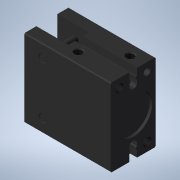
# Autodesk Inventor part: MCHA-20_(b)
Saved by Autodesk Inventor 2021 (Build 250183000, 183)
## iProperties
Created: 2025-07-26
Part Number: MCHA-20_(b)
Material: Generic
Catalog Web Link: www.cadenas.de
Description: MCHA-body-Grippers
Vendor: MINDMAN
Document SubType Name: Modeling
Designer: psAdmin
Manufacturer: MINDMAN
Mass: 44.4877 g
Surface Area: 130.835 cm^2
Volume: 44.4877 cm^3
Density: 1 g/cm^3
Appearance: PSOLRGB-175-175-175
Category: PARTsolutions
Company: MINDMAN
Title: MCHA-20_(b)
Author: Cadenas PARTsolutions
Comments: Grippers
PSOL_IDENT_0: {$CADENAS_DATA/23d-libs/mindman/end_of_arm_tooling/grippers/angular_gripper/mcha/mcha_body.prj},177
PSOL_IDENT_1: {VTYP=3D},{NB=MCHA-20_(b)},{LINA=MCHA-20_(b)},{NN=MCHA-body},{DATE=13.05.2025 08:42:05},{GEOMDATE=13
PSOL_IDENT_2: .05.2025 08:42:00},{VERSION=},{LINEID=30},{WBVAR=MODEL,SWITCH},{WBNUMERIC=}  {NB=MCHA-20_(b)},{LINA=
PSOL_IDENT_3: MCHA-20_(b)},{KT=DUMMY},{IDNR=MIN},{CODE=MCHA-20},{MODEL=MCHA},{TUBE=20},{A=22.0},{B=4},{C=10},{D=12
PSOL_IDENT_4: },{E=40.1},{F=18},{G=30},{H=8.0},{I=13.0},{J=25.0},{K=45},{L=25.0},{M=39.5},{N=32.5},{O=16.0},{P=19.
PSOL_IDENT_5: 0},{Q=50.0},{R=16},{S=26},{T=35},{UU=M5 x 8depth},{VV=M5 x 8depth},{WW=M5 x 12depth},{XX=M5 x 5depth
PSOL_IDENT_6: },{YY=M4},{Z=7},{ZZ=3.5},{A1=29.2},{B1=0.0},{C1=0.1},{A2=29.2},{B2=1.9},{C2=0.0},{SWITCH=},{XSWITCH=''
PSOL_IDENT_7: ,'Blank: without switch','+RCE','RCE : 2 wire (Reed switch)','+RDE','RDE : 2 wire (Non+contact)','+R
PSOL_IDENT_8: DE-D','RDE-D : 2 wire (Non+contact)','+RNE','RNE : 3 wire(NPN current sinking)','+RNEE','RNEE : 3 wi
PSOL_IDENT_9: re(NPN current sinking)','+RPE','RPE : 3 wire(PNP current sourcing)','+RPEE','RPEE : 3 wire(PNP curr
PSOL_IDENT_10: ent sourcing)'}
NB: MCHA-20_(b)
NN: MCHA-body
NT: Grippers
NBSYN: $CODE._(b)
LINA: MCHA-20_(b)
CATALOG: MINDMAN
MODEL: MCHA
TUBE: 20
A: 22
B: 4
C: 10
D: 12
E: 40.1
F: 18
G: 30
H: 8
I: 13
J: 25
K: 45
L: 25
M: 39.5
N: 32.5
O: 16
P: 19
Q: 50
R: 16
S: 26
T: 35
UU: M5 x 8depth
VV: M5 x 8depth
WW: M5 x 12depth
XX: M5 x 5depth
YY: M4
Z: 7
ZZ: 3.5
A1: 29.2
B1: 0
C1: 0.1
A2: 29.2
B2: 1.9
C2: 0
SWITCH: Blank: without switch
SUPPLIER: MINDMAN
ARTICLENO: MCHA-20_(b)
BOMINFO: MCHA-20_(b)
CREATOR: CADENAS GmbH
Autodesk Inventor part; units mm, degrees
sketch "Sketch_1" plane through (0, 0, 0) normal (1, 0, 0) x (0, 1, 0)
  line L0 (-22, 13) -> (-22.5, 12.5)
  line L1 (-22.5, 12.5) -> (-22.5, 2.25)
  line L2 (-22.5, 2.25) -> (-18.5, 2.25)
  line L3 (-18.5, 2.25) -> (-18.5, 1.9)
  arc A0 (-18.5, 1.9) -> (-18.3, 1.7) centre (-18.3, 1.9) ccw
  line L4 (-18.3, 1.7) -> (-17, 1.7)
  line L5 (-17, 1.7) -> (-16.5, 2.15)
  line L6 (-16.5, 2.15) -> (-14.7, 2.15)
  arc A1 (-13, 0.45) -> (-14.7, 2.15) centre (-14.7, 0.45) ccw
  line L7 (-13, 0.45) -> (-13, -0.45)
  arc A2 (-14.7, -2.15) -> (-13, -0.45) centre (-14.7, -0.45) ccw
  line L8 (-14.7, -2.15) -> (-16.5, -2.15)
  line L9 (-16.5, -2.15) -> (-17, -1.7)
  line L10 (-17, -1.7) -> (-18.3, -1.7)
  arc A3 (-18.3, -1.7) -> (-18.5, -1.9) centre (-18.3, -1.9) ccw
  line L11 (-18.5, -1.9) -> (-18.5, -2.25)
  line L12 (-18.5, -2.25) -> (-22.5, -2.25)
  line L13 (-22.5, -2.25) -> (-22.5, -12.5)
  line L14 (-22.5, -12.5) -> (-22, -13)
  line L15 (-22, -13) -> (22, -13)
  line L16 (22, -13) -> (22.5, -12.5)
  line L17 (22.5, -12.5) -> (22.5, -2.25)
  line L18 (22.5, -2.25) -> (18.5, -2.25)
  line L19 (18.5, -2.25) -> (18.5, -1.9)
  arc A4 (18.5, -1.9) -> (18.3, -1.7) centre (18.3, -1.9) ccw
  line L20 (18.3, -1.7) -> (17, -1.7)
  line L21 (17, -1.7) -> (16.5, -2.15)
  line L22 (16.5, -2.15) -> (14.7, -2.15)
  arc A5 (13, -0.45) -> (14.7, -2.15) centre (14.7, -0.45) ccw
  line L23 (13, -0.45) -> (13, 0.45)
  arc A6 (14.7, 2.15) -> (13, 0.45) centre (14.7, 0.45) ccw
  line L24 (14.7, 2.15) -> (16.5, 2.15)
  line L25 (16.5, 2.15) -> (17, 1.7)
  line L26 (17, 1.7) -> (18.3, 1.7)
  arc A7 (18.3, 1.7) -> (18.5, 1.9) centre (18.3, 1.9) ccw
  line L27 (18.5, 1.9) -> (18.5, 2.25)
  line L28 (18.5, 2.25) -> (22.5, 2.25)
  line L29 (22.5, 2.25) -> (22.5, 12.5)
  line L30 (22.5, 12.5) -> (22, 13)
  line L31 (22, 13) -> (-22, 13)
  constraints: 64 end point, 16 point on circle, 8 centre point
extrude "Extrusion1" add sketch "Sketch_1" along normal blind 50
sketch "Sketch2" plane through (50, 0, 0) normal (1, 0, 0) x (0, 0, -1)
  point P0 (0, 0)
hole "Hole1" at (50, 0, 0) direction (-1, 0, 0) diameter 22 depth 1.5
sketch "Sketch3" plane through (50, 0, 0) normal (1, 0, 0) x (0, 0, -1)
  point P0 (8, 17.5)
hole "Hole2" at (50, 17.5, -8) direction (-1, 0, 0) diameter 4 depth 4
sketch "Sketch_3" plane through (0, 0, 0) normal (0, 1, 0) x (-1, 0, 0)
  line L0 (0, 6.05) -> (-18.5, 6.05)
  line L1 (-18.5, 6.05) -> (-18.5, -6.05)
  line L2 (-18.5, -6.05) -> (0, -6.05)
  line L3 (0, -6.05) -> (0, 6.05)
  constraints: 8 end point
extrude "Extrusion2" cut sketch "Sketch_3" along normal mid plane 60
sketch "Sketch5" plane through (50, 0, 0) normal (1, 0, 0) x (0, 0, -1)
  point P0 (8, -17.5)
hole "Hole3" at (50, -17.5, -8) direction (-1, 0, 0) diameter 4.134 depth 11 tip angle 120 countersink diameter 5 countersink angle 90 thread size "M5x0.8" class "6H" standard "ISO Metric profile"
sketch "Sketch6" plane through (50, 0, 0) normal (1, 0, 0) x (0, 0, -1)
  point P0 (-8, 17.5)
hole "Hole4" at (50, 17.5, 8) direction (-1, 0, 0) diameter 4.134 depth 11 tip angle 120 countersink diameter 5 countersink angle 90 thread size "M5x0.8" class "6H" standard "ISO Metric profile"
sketch "Sketch_6" plane through (0, 0, 6.5) normal (0, 0, 1) x (1, 0, 0)
  line L0 (25, 6.3066) -> (25, 22.5)
  line L1 (25, 22.5) -> (27.5, 22.5)
  line L2 (27.5, 22.5) -> (27.067, 22.067)
  line L3 (27.067, 22.067) -> (27.067, 15.5)
  line L4 (27.067, 15.5) -> (25.75, 14.7396)
  line L5 (25.75, 14.7396) -> (25.75, 6.7396)
  line L6 (25.75, 6.7396) -> (25, 6.3066)
  line L7 (25, 6.3066) -> (25, 22.5)
  constraints: 16 end point
revolve "Revolution1" cut sketch "Sketch_6" angle 360 about axis through (25, 6.3066, 6.5) along (0, -1, 0)
thread "Thread1" size "M5x0.8" class "6H" standard "ISO Metric profile" length 4.567
sketch "Sketch_7" plane through (0, 0, -6.5) normal (0, 0, 1) x (1, 0, 0)
  line L0 (42, 6.3066) -> (42, 22.5)
  line L1 (42, 22.5) -> (44.5, 22.5)
  line L2 (44.5, 22.5) -> (44.067, 22.067)
  line L3 (44.067, 22.067) -> (44.067, 15.5)
  line L4 (44.067, 15.5) -> (42.75, 14.7396)
  line L5 (42.75, 14.7396) -> (42.75, 6.7396)
  line L6 (42.75, 6.7396) -> (42, 6.3066)
  line L7 (42, 6.3066) -> (42, 22.5)
  constraints: 16 end point
revolve "Revolution2" cut sketch "Sketch_7" angle 360 about axis through (42, 6.3066, -6.5) along (0, -1, 0)
thread "Thread2" size "M5x0.8" class "6H" standard "ISO Metric profile" length 4.567
sketch "Sketch9" plane through (0, -22.5, 12.5) normal (0, -1, 0) x (1, 0, 0)
  point P0 (31, -4.5)
hole "Hole5" at (31, -22.5, 8) direction (0, 1, 0) diameter 4.134 depth 11 tip angle 120 countersink diameter 5 countersink angle 90 thread size "M5x0.8" class "6H" standard "ISO Metric profile"
sketch "Sketch10" plane through (0, -22.5, -12.5) normal (0, -1, 0) x (1, 0, 0)
  point P0 (31, 4.5)
hole "Hole6" at (31, -22.5, -8) direction (0, 1, 0) diameter 4.134 depth 11 tip angle 120 countersink diameter 5 countersink angle 90 thread size "M5x0.8" class "6H" standard "ISO Metric profile"
sketch "Sketch11" plane through (0, -22, -13) normal (0, 0, -1) x (-1, 0, 0)
  point P0 (-25, 7)
hole "Hole7" at (25, -15, -13) direction (0, 0, 1) diameter 4.134 depth 12 tip angle 120 countersink diameter 5 countersink angle 90 thread size "M5x0.8" class "6H" standard "ISO Metric profile"
sketch "Sketch12" plane through (0, -22, -13) normal (0, 0, -1) x (-1, 0, 0)
  point P0 (-25, 37)
hole "Hole8" at (25, 15, -13) direction (0, 0, 1) diameter 4.134 depth 12 tip angle 120 countersink diameter 5 countersink angle 90 thread size "M5x0.8" class "6H" standard "ISO Metric profile"
sketch "Sketch_14" plane through (0, 15, 0) normal (0, 1, 0) x (1, 0, 0)
  line L0 (10.5, -13) -> (10.5, 13)
  line L1 (10.5, 13) -> (12.7, 13)
  line L2 (12.7, 13) -> (12.5, 12.8)
  line L3 (12.5, 12.8) -> (12.5, -12.8)
  line L4 (12.5, -12.8) -> (12.7, -13)
  line L5 (12.7, -13) -> (10.5, -13)
  line L6 (10.5, -13) -> (10.5, 13)
  constraints: 14 end point
revolve "Revolution3" cut sketch "Sketch_14" angle 360 about axis through (10.5, 15, 13) along (0, 0, 1)
sketch "Sketch_15" plane through (0, -15, 0) normal (0, 1, 0) x (1, 0, 0)
  line L0 (10.5, -13) -> (10.5, 13)
  line L1 (10.5, 13) -> (12.7, 13)
  line L2 (12.7, 13) -> (12.5, 12.8)
  line L3 (12.5, 12.8) -> (12.5, -12.8)
  line L4 (12.5, -12.8) -> (12.7, -13)
  line L5 (12.7, -13) -> (10.5, -13)
  line L6 (10.5, -13) -> (10.5, 13)
  constraints: 14 end point
revolve "Revolution4" cut sketch "Sketch_15" angle 360 about axis through (10.5, -15, 13) along (0, 0, 1)
sketch "Sketch_20" plane through (10.5, 0, 0) normal (1, 0, 0) x (0, 0, -1)
  line L0 (-12.9, 15) -> (12.9, 15)
  line L1 (12.9, 15) -> (12.9, 13)
  line L2 (12.9, 13) -> (-12.9, 13)
  line L3 (-12.9, 13) -> (-12.9, 15)
  line L4 (-12.9, 15) -> (12.9, 15)
  constraints: 10 end point
revolve "Revolution5" add sketch "Sketch_20" angle 360 about axis through (10.5, 15, 12.9) along (0, 0, 1)
sketch "Sketch_21" plane through (10.5, 0, 0) normal (1, 0, 0) x (0, 0, -1)
  line L0 (-12.9, -15) -> (12.9, -15)
  line L1 (12.9, -15) -> (12.9, -17)
  line L2 (12.9, -17) -> (-12.9, -17)
  line L3 (-12.9, -17) -> (-12.9, -15)
  line L4 (-12.9, -15) -> (12.9, -15)
  constraints: 10 end point
revolve "Revolution6" add sketch "Sketch_21" angle 360 about axis through (10.5, -15, 12.9) along (0, 0, 1)
ref_plane "dummy_XY" through (0, 0, 0) normal (1, 0, 0) x (0, 0, -1)
ref_plane "dummy_YZ" through (0, 0, 0) normal (0, 0, -1) x (0, 1, 0)
ref_plane "dummy_ZX" through (0, 0, 0) normal (0, 1, 0) x (1, 0, 0)
ref_plane "grip_XY" through (10.5, 15, 0) normal (0, 0, 1) x (1, 0, 0)
ref_plane "grip_YZ" through (10.5, 15, 0) normal (1, 0, 0) x (0, 1, 0)
ref_plane "grip_ZX" through (10.5, 15, 0) normal (0, 1, 0) x (0, 0, 1)
ref_plane "grip1_XY" through (10.5, -15, 0) normal (0, 0, 1) x (1, 0, 0)
ref_plane "grip1_YZ" through (10.5, -15, 0) normal (1, 0, 0) x (0, 1, 0)
ref_plane "grip1_ZX" through (10.5, -15, 0) normal (0, 1, 0) x (0, 0, 1)
ref_plane "switch_XY" through (20.8, 13, 0) normal (-1, 0, 0) x (0, 0, -1)
ref_plane "switch_YZ" through (20.8, 13, 0) normal (0, 0, -1) x (0, -1, 0)
ref_plane "switch_ZX" through (20.8, 13, 0) normal (0, -1, 0) x (-1, 0, 0)
ref_plane "switch2_XY" through (26.1, -13, 0) normal (-1, 0, 0) x (0, 0, -1)
ref_plane "switch2_YZ" through (26.1, -13, 0) normal (0, 0, -1) x (0, -1, 0)
ref_plane "switch2_ZX" through (26.1, -13, 0) normal (0, -1, 0) x (-1, 0, 0)
body "Solid1"
